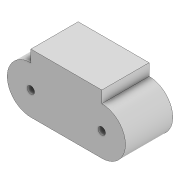
# Autodesk Inventor part: Part7
Saved by Autodesk Inventor 2022 (Build 260153000, 153)
## iProperties
Created: 2022-08-27
Part Number: Part7
Material: Generic
Document SubType Name: Modeling
Designer: dell
Density: 1 g/cm^3
Appearance: Default
Author: dell
Autodesk Inventor part; units mm, degrees
ref_plane "YZ Plane" through (0, 0, 0) normal (1, 0, 0) x (0, 1, 0)
ref_plane "XZ Plane" through (0, 0, 0) normal (0, 1, 0) x (-1, 0, 0)
ref_plane "XY Plane" through (0, 0, 0) normal (0, 0, 1) x (1, 0, 0)
sketch "Sketch1" plane through (0, 0, 0) normal (0, 0, 1) x (1, 0, 0)
  line L0 (0, 0) -> (-30, 0) construction
  line L1 (0, 10) -> (-30, 10)
  line L2 (-30, -10) -> (0, -10)
  arc A0 (0, -10) -> (0, 10) centre (0, 0) ccw
  arc A1 (-30, 10) -> (-30, -10) centre (-30, 0) ccw
  circle A2 centre (-30, 0) radius 1.55
  circle A3 centre (0, 0) radius 1.55
  line L3 (-30, 10) -> (0, 10)
  line L4 (0, 10) -> (0, 15)
  line L5 (0, 15) -> (-30, 15)
  line L6 (-30, 15) -> (-30, 10)
  point P0 (-15, 0)
  dimension "d0" = 20
  dimension "d1" = 30
  dimension "d2" = 3.1
  dimension "d3" = 3.1
  dimension "d7" = 5
  constraints: 16 end point, 4 centre point, 4 equal length, 4 point on circle, 4 tangent, 2 coincident, 1 horizontal, 1 midpoint, 1 perpendicular
  measures "d0" diameter of A1
  measures "d1" distance of L0.end L0.start
  measures "d2" diameter of A2
  measures "d3" diameter of A3
  measures "d7" distance of L4.end L1.start
extrude "Extrusion1" add sketch "Sketch1" along normal blind 20
body "Solid1"
